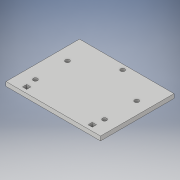
# Autodesk Inventor part: baseforclamp
Saved by Autodesk Inventor 2019 (Build 230136000, 136)
## iProperties
Created: 2020-02-26
Part Number: baseforclamp
Material: Generic
Document SubType Name: Modeling
Designer: Hp
Density: 1 g/cm^3
Appearance: Default
Author: Hp
Autodesk Inventor part; units mm, degrees
ref_plane "YZ Plane" through (0, 0, 0) normal (1, 0, 0) x (0, 1, 0)
ref_plane "XZ Plane" through (0, 0, 0) normal (0, 1, 0) x (-1, 0, 0)
ref_plane "XY Plane" through (0, 0, 0) normal (0, 0, 1) x (1, 0, 0)
sketch "Sketch1" plane through (0, 0, 0) normal (0, 1, 0) x (-1, 0, 0)
  line L0 (22.9947, 17.3637) -> (-22.0053, 17.3637)
  line L1 (-22.0053, 17.3637) -> (-22.0053, -17.6363)
  line L2 (-22.0053, -17.6363) -> (22.9947, -17.6363)
  line L3 (22.9947, -17.6363) -> (22.9947, 17.3637)
  circle A0 centre (16.8206, -5.7512) radius 1
  circle A1 centre (-16.1167, -5.7512) radius 1
  circle A2 centre (-16.1167, 9.54) radius 1
  circle A3 centre (16.8206, 9.54) radius 1
  line L4 (16.8206, 15.6616) -> (14.8206, 15.6616)
  line L5 (14.8206, 15.6616) -> (14.8206, 13.6616)
  line L6 (14.8206, 13.6616) -> (16.8206, 13.6616)
  line L7 (16.8206, 13.6616) -> (16.8206, 15.6616)
  line L8 (-16.3896, 13.6616) -> (-14.3896, 13.6616)
  line L9 (-14.3896, 13.6616) -> (-14.3896, 15.6616)
  line L10 (-14.3896, 15.6616) -> (-16.3896, 15.6616)
  line L11 (-16.3896, 15.6616) -> (-16.3896, 13.6616)
  line L12 (14.8206, 13.6616) -> (-14.3896, 13.6616)
  circle A4 centre (0.2155, -14.9426) radius 1
  point P0 (0, 0)
  dimension "d0" = 45
  dimension "d1" = 35
  dimension "d2" = 2
  dimension "d3" = 2
  dimension "d4" = 2
  dimension "d5" = 2
  dimension "d6" = 2
  dimension "d7" = 2
  dimension "d8" = 2
  dimension "d9" = 2
  dimension "d10" = 29.2102
  dimension "d13" = 2
  constraints: 26 end point, 6 parallel, 5 centre point, 3 horizontal, 3 perpendicular, 1 point on line
  measures "d0" distance of L2.end L1.end
  measures "d1" distance of L1.end L0.end
  measures "d2" diameter of A0
  measures "d3" diameter of A1
  measures "d4" diameter of A2
  measures "d5" diameter of A3
  measures "d6" distance of L6.end L5.end
  measures "d7" distance of L5.end L4.end
  measures "d8" distance of L10.end L9.end
  measures "d9" distance of L9.end L8.end
  measures "d10" distance of L5.end L12.end
  measures "d13" diameter of A4
extrude "Extrusion1" add sketch "Sketch1" along normal blind 2 contours L3 L2 L1 L0 | A4
sketch "Sketch2" plane through (0, 2, 0) normal (0, 1, 0) x (1, 0, 0)
  circle A0 centre (0, 15.1758) radius 1
  point P0 (0, 0)
  dimension "d14" = 2
  constraints: 1 centre point
  measures "d14" diameter of A0
extrude "Extrusion2" cut sketch "Sketch2" against normal blind 10
body "Solid1"
